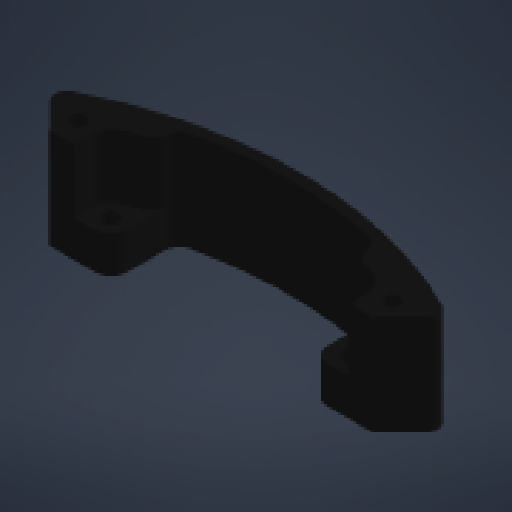
# Autodesk Inventor part: Side Wall
Saved by Autodesk Inventor 2026.1 (Build 301233020, 233B)
## iProperties
Created: 2026-04-03
Part Number: Side Wall
Material: Generic
Document SubType Name: Modeling
Designer: Bahaa
Density: 1 g/cm^3
Appearance: Default(1)
Mass: 18.3658 g
Surface Area: 84.1643 cm^2
Volume: 18.3658 cm^3
Author: Bahaa
Autodesk Inventor part; units mm, degrees
ref_plane "YZ Plane" through (0, 0, 0) normal (1, 0, 0) x (0, 1, 0)
ref_plane "XZ Plane" through (0, 0, 0) normal (0, 1, 0) x (-1, 0, 0)
ref_plane "XY Plane" through (0, 0, 0) normal (0, 0, 1) x (1, 0, 0)
sketch "Sketch1" plane through (0, 0, 0) normal (0, 0, 1) x (1, 0, 0)
  circle A0 centre (40.84062, 22.799513) radius 1.6
  circle A1 centre (-40.84062, 22.799513) radius 1.6
  line L0 (-42.160334, 16.778698) -> (-35.890873, 16.778698)
  line L1 (-35.890873, 16.778698) -> (-35.890873, 21.054791)
  arc A2 (-31.809004, 26.739927) -> (-35.890873, 21.054791) centre (-29.890873, 21.054791) ccw
  arc A3 (31.809004, 26.739927) -> (-31.809004, 26.739927) centre (0, -67.538582) ccw
  arc A4 (35.890873, 21.054791) -> (31.809004, 26.739927) centre (29.890873, 21.054791) ccw
  line L2 (35.890873, 21.054791) -> (35.890873, 16.778698)
  line L3 (35.890873, 16.778698) -> (42.160334, 16.778698)
  arc A5 (42.769553, 17.657377) -> (42.160334, 16.778698) centre (44.890873, 15.536057) ccw
  line L4 (42.769553, 17.657377) -> (48.898315, 23.78614)
  arc A6 (48.898315, 23.78614) -> (48.119875, 28.590121) centre (46.776995, 25.90746) ccw
  arc A7 (48.119875, 28.590121) -> (-48.119875, 28.590121) centre (0, -67.538582) ccw
  arc A8 (-48.119875, 28.590121) -> (-48.898315, 23.78614) centre (-46.776995, 25.90746) ccw
  line L5 (-48.898315, 23.78614) -> (-42.769553, 17.657377)
  arc A9 (-42.160334, 16.778698) -> (-42.769553, 17.657377) centre (-44.890873, 15.536057) ccw
  line L6 (-26.109127, 29.144138) -> (-35.890873, 29.144138) construction
  line L7 (-35.890873, 29.144138) -> (-35.890873, 16.778698) construction
  line L8 (-35.890873, 16.778698) -> (-26.109127, 16.778698)
  line L9 (-26.109127, 16.778698) -> (-26.109127, 29.144138)
  line L10 (-26.109127, 29.144138) -> (-35.890873, 16.778698) construction
  line L11 (-35.890873, 29.144138) -> (-26.109127, 16.778698) construction
  line L12 (-31, 29.144138) -> (-31, 22.961418) construction
  line L13 (-31, 21.461418) -> (-31, 22.961418) construction
  line L14 (-31, 21.461418) -> (-31, 16.778698) construction
  line L15 (0, 31.961418) -> (0, 39.961418) construction
  line L16 (35.890873, 16.778698) -> (35.890873, 21.054791)
  arc A10 (35.890873, 21.054791) -> (31.809004, 26.739927) centre (29.890873, 21.054791) ccw
  line L17 (26.109127, 29.144138) -> (35.890873, 29.144138) construction
  line L18 (35.890873, 29.144138) -> (35.890873, 16.778698) construction
  line L19 (35.890873, 16.778698) -> (26.109127, 16.778698)
  line L20 (26.109127, 16.778698) -> (26.109127, 29.144138)
  line L21 (26.109127, 29.144138) -> (35.890873, 16.778698) construction
  line L22 (35.890873, 29.144138) -> (26.109127, 16.778698) construction
  line L23 (31, 29.144138) -> (31, 22.961418) construction
  line L24 (31, 21.461418) -> (31, 22.961418) construction
  line L25 (31, 21.461418) -> (31, 16.778698) construction
  arc A11 (-32.768069, 29.582495) -> (-38.890873, 21.054791) centre (-29.890873, 21.054791) ccw
  line L26 (-38.890873, 21.054791) -> (-38.890873, 19.778698)
  line L27 (-38.890873, 19.778698) -> (-40.648232, 19.778698)
  arc A12 (-40.648232, 19.778698) -> (-40.648232, 19.778698) centre (-44.890873, 15.536057) ccw
  line L28 (-40.648232, 19.778698) -> (-46.776995, 25.90746)
  arc A13 (-46.776995, 25.90746) -> (-46.776995, 25.90746) centre (-46.776995, 25.90746) ccw
  arc A14 (46.776995, 25.90746) -> (-46.776995, 25.90746) centre (0, -67.538582) ccw
  arc A15 (46.776995, 25.90746) -> (46.776995, 25.90746) centre (46.776995, 25.90746) ccw
  line L29 (46.776995, 25.90746) -> (40.648232, 19.778698)
  arc A16 (40.648232, 19.778698) -> (40.648232, 19.778698) centre (44.890873, 15.536057) ccw
  line L30 (40.648232, 19.778698) -> (38.890873, 19.778698)
  line L31 (38.890873, 19.778698) -> (38.890873, 21.054791)
  arc A17 (38.890873, 21.054791) -> (32.768069, 29.582495) centre (29.890873, 21.054791) ccw
  arc A18 (32.768069, 29.582495) -> (-32.768069, 29.582495) centre (0, -67.538582) ccw
  line L32 (-26.109127, 29.144138) -> (-26.109127, 33.647205)
  line L33 (26.109127, 29.144138) -> (26.109127, 33.647205)
  point P0 (0, 0)
  point P1 (-26.109127, 28.474768)
  point P2 (-31, 22.961418)
  point P3 (31, 22.961418)
  point P4 (26.109127, 28.474768)
  point P5 (-26.109127, 31.580354)
  point P6 (26.109127, 31.580354)
  point P7 (26.109127, 33.647205)
  dimension "d33" = 31
  dimension "d34" = 9
  dimension "d35" = 1.5
  dimension "d50" = 2
  constraints: 56 end point, 17 point on circle, 10 symmetric about line, 9 centre point, 4 coincident with centre, 4 midpoint, 2 coincident, 2 parallel, 1 collinear, 1 horizontal, 1 perpendicular, 1 point on line, 1 vertical, 14 other
  measures "d33" horizontal distance of point (-31, 22.961) L15.start
  measures "d34" vertical distance of L15.start point (-31, 22.961)
  measures "d35" distance of L13.start L12.end
  measures "d50" radial gap between concentric circles of A18 A14
sketch "Sketch1 outline for Extrusion1" plane through (0, 0, 0) normal (0, 0, 1) x (1, 0, 0)
  arc A0 (-26.109127, 33.647205) -> (26.109127, 33.647205) centre (0, -67.538582) cw
  line L0 (26.109127, 33.647205) -> (26.109127, 16.778698)
  line L1 (26.109127, 16.778698) -> (42.160334, 16.778698)
  arc A1 (42.160334, 16.778698) -> (42.769553, 17.657377) centre (44.890873, 15.536057) cw
  line L2 (42.769553, 17.657377) -> (48.898315, 23.78614)
  arc A2 (48.898315, 23.78614) -> (48.119875, 28.590121) centre (46.776995, 25.90746) ccw
  arc A3 (48.119875, 28.590121) -> (-48.119875, 28.590121) centre (0, -67.538582) ccw
  arc A4 (-48.119875, 28.590121) -> (-48.898315, 23.78614) centre (-46.776995, 25.90746) ccw
  line L3 (-48.898315, 23.78614) -> (-42.769553, 17.657377)
  arc A5 (-42.769553, 17.657377) -> (-42.160334, 16.778698) centre (-44.890873, 15.536057) cw
  line L4 (-42.160334, 16.778698) -> (-26.109127, 16.778698)
  line L5 (-26.109127, 16.778698) -> (-26.109127, 33.647205)
extrude "Extrusion1" add sketch "Sketch1 outline for Extrusion1" along normal blind 26
sketch "Sketch2" plane through (0, 0, 26) normal (0, 0, 1) x (1, 0, 0)
  point P0 (0, 0)
  point P1 (-40.84062, 22.799513)
  point P2 (40.84062, 22.799513)
hole "Hole1" at (-40.84062, 22.799513, 26) at (40.84062, 22.799513, 26) direction (0, 0, -1) diameter 4.2 depth 6
sketch "Sketch3" plane through (0, 0, 0) normal (0, 0, -1) x (-1, 0, 0)
  point P0 (0, 0)
  point P1 (40.84062, 22.799513)
  point P2 (-40.84062, 22.799513)
hole "Hole2" at (-40.84062, 22.799513, 0) at (40.84062, 22.799513, 0) direction (0, 0, 1) diameter 4.2 depth 6
sketch "Sketch4" plane through (0, 0, 26) normal (0, 0, -1) x (-1, 0, 0)
  arc A0 (35.890873, 21.054791) -> (31.809004, 26.739927) centre (29.890873, 21.054791) ccw
  arc A1 (31.809004, 26.739927) -> (-31.809004, 26.739927) centre (0, -67.538582) ccw
  line L0 (35.890873, 29.144138) -> (35.890873, 16.778698) construction
  line L1 (35.890873, 16.778698) -> (35.890873, 21.054791)
  line L2 (35.890873, 16.778698) -> (26.109127, 16.778698)
  line L3 (26.109127, 16.778698) -> (26.109127, 29.144138)
  line L4 (-26.109127, 28.474768) -> (-26.109127, 16.778698)
  line L5 (-35.890873, 16.778698) -> (-26.109127, 16.778698)
  line L6 (-35.890873, 21.054791) -> (-35.890873, 16.778698)
  arc A2 (-31.809004, 26.739927) -> (-35.890873, 21.054791) centre (-29.890873, 21.054791) ccw
  point P0 (0, 0)
  point P1 (26.109127, 28.474768)
extrude "Extrusion2" cut sketch "Sketch4" along normal blind 17 from surface at 0
fillet "Fillet1" radius 4 6 edges at (-26.1091, 16.7787, 4.5) (26.1091, 16.7787, 4.5) (-26.1091, 33.6472, 13) (26.1091, 33.6472, 13) (-26.1091, 28.4748, 17.5) (26.1091, 28.4748, 17.5)
sketch "Sketch5" plane through (-35.890873, 16.778698, 9) normal (0, 0, 1) x (1, 0, 0)
  point P0 (35.890873, -16.778698)
  point P1 (4.890873, 4.68272)
  point P2 (66.890873, 4.68272)
hole "Hole3" at (-31, 21.461418, 9) at (31, 21.461418, 9) direction (0, 0, -1) diameter 4.2 depth 6
body "Solid1"
